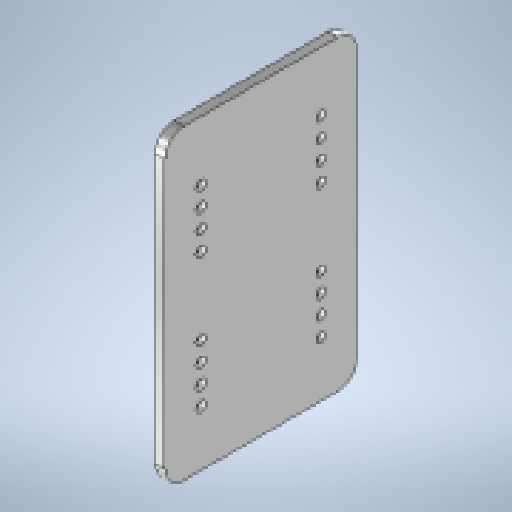
# Autodesk Inventor part: Ramp
Saved by Autodesk Inventor 2023.2 (Build 272271000, 271)
## iProperties
Created: 2024-02-17
Part Number: Ramp
Material: Aluminum 6061
Document SubType Name: Modeling
Designer: Nathan Cai
Density: 2.7 g/cm^3
Appearance: Aluminum - Flat
Mass: 47.8529 g
Surface Area: 126.839 cm^2
Volume: 17.7233 cm^3
Author: Nathan Cai
Autodesk Inventor part; units mm, degrees
ref_plane "YZ Plane" through (0, 0, 0) normal (1, 0, 0) x (0, 1, 0)
ref_plane "XZ Plane" through (0, 0, 0) normal (0, 1, 0) x (-1, 0, 0)
ref_plane "XY Plane" through (0, 0, 0) normal (0, 0, 1) x (1, 0, 0)
sketch "Sketch1" plane through (0, 0, 0) normal (1, 0, 0) x (0, 1, 0)
  line L0 (50.8, 28.575) -> (-50.8, 28.575)
  line L1 (-50.8, 28.575) -> (-50.8, -28.575)
  line L2 (-50.8, -28.575) -> (50.8, -28.575)
  line L3 (50.8, -28.575) -> (50.8, 28.575)
  line L4 (50.8, 28.575) -> (-50.8, -28.575) construction
  line L5 (-50.8, 28.575) -> (50.8, -28.575) construction
  point P0 (0, 0)
  dimension "d0" = 101.6
  dimension "d1" = 57.15
  constraints: 12 end point, 2 midpoint, 2 parallel, 1 horizontal, 1 perpendicular
  measures "d0" distance of L2.end L1.end
  measures "d1" distance of L1.end L0.end
extrude "Extrusion1" add sketch "Sketch1" along normal blind 3.175
sketch "Sketch2" plane through (0, 0, 0) normal (-1, 0, 0) x (0, 0, 1)
  point P0 (19.8437, 30.9563)
  point P1 (19.8437, 24.6063)
  point P2 (19.8437, 18.2563)
  point P3 (19.8437, 11.9063)
  point P4 (19.8437, -13.4937)
  point P5 (19.8437, -19.8437)
  point P6 (19.8437, -26.1937)
  point P7 (19.8437, -32.5437)
  point P8 (-19.8438, -32.5437)
  point P9 (-19.8438, -26.1937)
  point P10 (-19.8438, -19.8437)
  point P11 (-19.8438, -13.4937)
  point P12 (-19.8438, 11.9063)
  point P13 (-19.8438, 18.2563)
  point P14 (-19.8438, 24.6063)
  point P15 (-19.8438, 30.9563)
hole "Hole1" at (0, 30.9563, 19.8437) at (0, 24.6063, 19.8437) at (0, 18.2563, 19.8437) at (0, 11.9063, 19.8437) at (0, -13.4937, 19.8437) at (0, -19.8437, 19.8437) at (0, -26.1937, 19.8437) at (0, -32.5437, 19.8437) at (0, -32.5437, -19.8438) at (0, -26.1937, -19.8438) at (0, -19.8437, -19.8438) at (0, -13.4937, -19.8438) at (0, 11.9063, -19.8438) at (0, 18.2563, -19.8438) at (0, 24.6063, -19.8438) at (0, 30.9563, -19.8438) direction (1, 0, 0) diameter 3.2639 end through all countersink diameter 5.715 countersink angle 82
body "Solid1"
